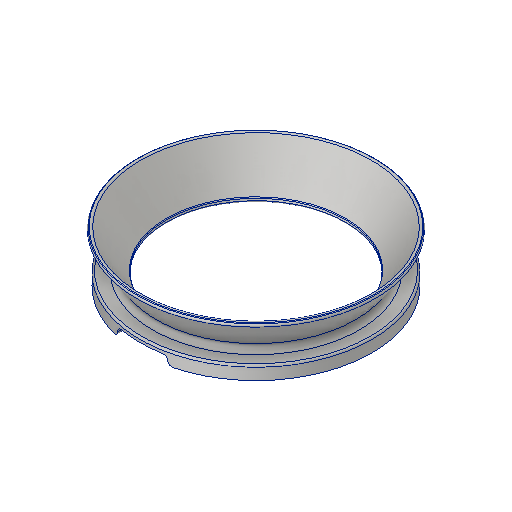
# Autodesk Inventor part: CNCM_ALU_Regolith_container_funnel
Saved by Autodesk Inventor 2025 (Build 290162010, 162A)
## iProperties
Created: 2018-09-18
Part Number: CNCM_ALU_Regolith_container_funnel
Material: Aluminum 6061
Document SubType Name: Modeling
Designer: Andrzej
Density: 2.7 g/cm^3
Appearance: Aluminum - Flat
Mass: 7.53054 g
Surface Area: 53.6258 cm^2
Volume: 2.78909 cm^3
Author: Andrzej
Autodesk Inventor part; units mm, degrees
ref_plane "YZ Plane" through (0, 0, 0) normal (1, 0, 0) x (0, 1, 0)
ref_plane "XZ Plane" through (0, 0, 0) normal (0, 1, 0) x (-1, 0, 0)
sketch "Sketch1" plane through (0, 0, 0) normal (0, 0, 1) x (1, 0, 0)
  line L0 (-20, 1.125) -> (-26, 1.125)
  line L1 (-26, 1.125) -> (-26, -1.875)
  line L2 (-26, -1.875) -> (-25, -1.875)
  line L3 (-25, -1.875) -> (-25, 0.125)
  line L4 (-25, 0.125) -> (-20, 0.125)
  line L5 (-20, 0.125) -> (-20, 1.125)
  line L6 (-21.2184, 1.125) -> (-26.9314, 9.3324)
  line L7 (-26.9314, 9.3324) -> (-26.1107, 9.9037)
  line L8 (-26.1107, 9.9037) -> (-20, 1.125)
  line L9 (0, -4.2307) -> (0, 12.2594) projected
  point P0 (0, 0)
  dimension "d0" = 1
  dimension "d1" = 1
  dimension "d2" = 26
  dimension "d3" = 25
  dimension "d4" = 20
  dimension "d5" = 10
  dimension "d6" = 1
  dimension "d7" = 2
  constraints: 18 end point, 5 perpendicular, 1 horizontal, 1 parallel, 1 point on line, 1 vertical
  measures "d0" distance between parallel lines of L3 L1
  measures "d1" distance between parallel lines of L0 L4
  measures "d2" distance from line of point (0, 0) L1
  measures "d3" distance from line of point (0, 0) L3
  measures "d4" distance from line of point (0, 0) L5
  measures "d5" distance of L6.start L6.end
  measures "d6" distance between parallel lines of L6 L8
  measures "d7" distance between parallel lines of L2 L4
revolve "Revolution1" add sketch "Sketch1" angle 360 about axis through (0, -10, 0) along (0, 1, 0)
fillet "Fillet1" radius 1 1 edges at (21.2184, 1.125, 0)
fillet "Fillet1" radius 0.4 5 edges at (26.1107, 9.9037, 0) (26.9314, 9.3324, 0) (20, 1.125, 0) (20, 0.125, 0) (26, 1.125, 0)
ref_plane "Work Plane1" through (0, 0, 30) normal (0, 0, 1) x (1, 0, 0)
sketch "Sketch2" plane through (0, 0, 30) normal (0, 0, 1) x (1, 0, 0)
  line L0 (25, 0.125) -> (-25, 0.125) projected
  line L1 (-5.6, 0.125) -> (5.6, 0.125)
  line L2 (5.6, 0.125) -> (5.6, -3.875)
  line L3 (5.6, -3.875) -> (-5.6, -3.875)
  line L4 (-5.6, -3.875) -> (-5.6, 0.125)
  point P0 (0, 0)
  dimension "d12" = 11.2
  dimension "d13" = 5.6
  dimension "d14" = 4
  constraints: 8 end point, 2 parallel, 1 horizontal, 1 perpendicular, 1 point on line
  measures "d12" distance of L2.end L3.end
  measures "d13" distance from line of L4 point (0, 0)
  measures "d14" distance of L3.end L1.start
extrude "Extrusion1" cut sketch "Sketch2" against normal blind 10
fillet "Fillet2" radius 1 4 edges at (-5.6, 0.125, 24.8772) (5.6, 0.125, 24.8772) (5.6, -1.875, 24.8772) (-5.6, -1.875, 24.8772)
equation "\"d13\" = 0.5 * d12"
body "Solid1"
